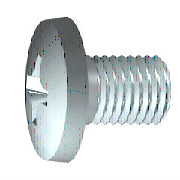
# Autodesk Inventor part: JIS B 1111 - M8x30
Saved by Autodesk Inventor 2022 (Build 260153000, 153)
## iProperties
Created: 2021-02-02
Part Number: JIS B 1111 - M8x30
Material: Сталь, мягкая
Description: Винты с низкой цилиндрической головкой
Document SubType Name: Modeling
Standard: JIS B 1111
Designer: Petrov Ivan
Standards Organization: JIS
Language: ru-RU
Size Designation: M8x30
Categories: <MemberInstance><Categories><Category DisplayName="Крепежные изделия" InternalName="e4da775c-781d-43d5-af7c-5136215cf5a6" Mnemonic="FSTN"><Category DisplayName="Болты  Винты" InternalName="536e6df0-f778-49ac-b2f2-25c71d2aa0b2" Mnemonic="SCRW"><CategoryParameter DisplayName="Обозначение номинального диаметра" InternalName="03caf894-eafd-4c09-a035-916ac084b87b" Mnemonic="nomdiadesig"/><CategoryParameter DisplayName="Номинальная длина" InternalName="238ecbaf-3e6c-45dd-aa95-4068c8e0fd02" Mnemonic="nomlen"/><CategoryParameter DisplayName="Обозначение резьбы" InternalName="586d5e89-370a-4089-914f-0110033585c7" Mnemonic="thrdesign"/><CategoryParameter DisplayName="Обозначение серии резьб" InternalName="87c5849c-b3a5-4c3e-9c9b-2feecef9be86" Mnemonic="thrserdsgn"/><CategoryParameter DisplayName="Номинальный диаметр" InternalName="8bbe3f8e-44cf-40a9-a251-3a6edc8168d6" Mnemonic="nomdia"/><CategoryParameter DisplayName="Тип резьбы" InternalName="b4bbb7bc-d6aa-4c9f-a9a9-4152b9f6fe49" Mnemonic="thrtype"/><CategoryParameter DisplayName="Шаг резьбы" InternalName="bb82302e-82d8-4176-8fc1-c5d7bb17d5ad" Mnemonic="pitch1"/><CategoryParameter DisplayName="Витков на единицу" InternalName="bdc6e7d2-ffd0-4d9c-a173-16b95ebb912d" Mnemonic="thrperunit1"/><CategoryParameter DisplayName="Класс резьбы" InternalName="ebc0d23b-2cc6-4d2a-b376-d52aae53bab6" Mnemonic="thrclss"/><Category DisplayName="С углублением под ключ" InternalName="55e06bf3-7e58-486c-bbdc-745fcc60664d" Mnemonic="CLSCRW"><CategoryParameter DisplayName="Диаметр стержня" InternalName="179dbae3-102f-48bb-85fe-1e3ecd34f7cc" Mnemonic="grpdia"/><CategoryParameter DisplayName="Длина резьбы" InternalName="3268731d-5f9a-4750-8b01-4a959c46fbf2" Mnemonic="thrlen"/><CategoryParameter DisplayName="Диаметр головки" InternalName="46177176-dbdd-4a1b-aefd-4c60c45016af" Mnemonic="headdia"/><CategoryParameter DisplayName="Длина стержня" InternalName="52eab69f-422f-4795-9995-175a1b827e67" Mnemonic="grplen"/><CategoryParameter DisplayName="Тип" InternalName="59a7e495-7a0c-4a5c-bdfd-c090c5f6e2db" Mnemonic="type"/><CategoryParameter DisplayName="Высота головки" InternalName="99c92c4c-4a02-4ebe-9e64-948fb169e19e" Mnemonic="headh"/></Category></Category></Category><Category DisplayName="ТипДанных" InternalName="23b78d0f-2648-40c6-8793-ca6db495c9e8" Mnemonic="DATATYPE"><CategoryParameter DisplayName="ОтображаемоеИмя" InternalName="05415f3d-3907-474b-a020-eb9d644f4cf3" Mnemonic="DISPLAYNAME"/><CategoryParameter DisplayName="Стандарт" InternalName="0c0a119c-1e12-4c84-803f-101930972f5e" Mnemonic="STANDARD"/><CategoryParameter DisplayName="Наименование" InternalName="13903e3d-64b1-4950-80da-f627842ea37f" Mnemonic="DESCRIPTION"/><CategoryParameter DisplayName="Обозначение" InternalName="2675968c-4ce5-49e0-a4f5-552d29089031" Mnemonic="DESIGNATION"/><CategoryParameter DisplayName="Строка по умолчанию" InternalName="2af9ec52-faaa-4026-b378-f9fa4afca842" Mnemonic="DEFAULTROW"/><CategoryParameter DisplayName="Имя папки" InternalName="3f06958e-8713-4116-9be7-ed6184ecc97b" Mnemonic="FOLDERNAME"/><CategoryParameter DisplayName="Указатель редакций" InternalName="45a75005-10b1-4dfc-8d6d-dfe629f0b93c" Mnemonic="REVISIONGUID"/><CategoryParameter DisplayName="ИмяФайла" InternalName="8b46a4cc-9585-4fed-90c3-899f57e09a73" Mnemonic="FILENAME"/><CategoryParameter DisplayName="ОргСтанд" InternalName="8f5914e1-4693-403f-8ab5-d37768198c9d" Mnemonic="STDSORG"/><CategoryParameter DisplayName="Версия семейства" InternalName="914462f6-6e19-4b14-ba84-155b9680b1d0" Mnemonic="FAMILYREVISION"/><CategoryParameter DisplayName="Редакция стандарта" InternalName="91d5a463-65c2-4fde-b823-3b7fea5e8e17" Mnemonic="STANDARDREVISION"/><CategoryParameter DisplayName="редакция элемента" InternalName="a65d44b9-392f-4f4f-857b-e4b3d54996fe" Mnemonic="MEMBERREVISION"/><CategoryParameter DisplayName="ФорматКлипа" InternalName="bc51e27b-3422-4e78-93ef-cec197ddf230" Mnemonic="CLIPFORMAT"/><CategoryParameter DisplayName="Изготовитель" InternalName="cd6c7a72-a28a-4e50-99a9-2c7f4e13e5ad" Mnemonic="MANUFACTURER"/><CategoryParameter DisplayName="ВнутреннееИмя" InternalName="cf1d0246-76d9-4b4a-8305-fa0409afb5c1" Mnemonic="INTERNALNAME"/><CategoryParameter DisplayName="Метрическая" InternalName="e2385c5b-1ea4-4823-96a8-8de651266ec3" Mnemonic="ISMETRIC"/><Category DisplayName="Деталь" InternalName="c0e0b642-3bcb-4cc8-9e80-f96d35c4afa4" Mnemonic="PART"><CategoryParameter DisplayName="Номер детали" InternalName="016b6077-bfbe-49bd-92c9-d8d59c39c941" Mnemonic="PARTNUMBER"/><CategoryParameter DisplayName="Инвентарный номер" InternalName="4dba7c1c-e26c-444e-836c-b08b433409a8" Mnemonic="STOCKNUMBER"/><CategoryParameter DisplayName="Ключ материала" InternalName="5c9a8adb-dd2b-4535-b97f-0a94a95fe41f" Mnemonic="MATERIALKEY"/><CategoryParameter DisplayName="Материал" InternalName="818a152a-d3c3-49ca-80ee-df7d91421b8e" Mnemonic="MATERIAL"/></Category></Category><Category DisplayName="Схема предыдущей версии DA" InternalName="924fff40-ddd0-4eff-ad42-30e3774ef79e" Mnemonic="LEGACYMAPDA"><CategoryParameter DisplayName="DACookie" InternalName="316934ee-8fe1-4c7a-9c36-f2d79e1add1a" Mnemonic="DACOOKIE"/></Category></Categories><FamilyTemplate Id="J11119"><FamilyTemplateParameters><FamilyTemplateParameter ObjectType="kUserParameterObject" ValueType="xs:double" Id="1" ObjectReferenceKey="NND"/><FamilyTemplateParameter ObjectType="kUserParameterObject" ValueType="xs:double" Id="2" ObjectReferenceKey="NLG"/><FamilyTemplateParameter ObjectType="kUserParameterObject" ValueType="xs:double" Id="3" ObjectReferenceKey="PTC"/><FamilyTemplateParameter ObjectType="kUserParameterObject" ValueType="xs:double" Id="4" ObjectReferenceKey="Dk"/><FamilyTemplateParameter ObjectType="kUserParameterObject" ValueType="xs:double" Id="5" ObjectReferenceKey="ParK"/><FamilyTemplateParameter ObjectType="kUserParameterObject" ValueType="xs:double" Id="6" ObjectReferenceKey="M"/><FamilyTemplateParameter ObjectType="kUserParameterObject" ValueType="xs:double" Id="7" ObjectReferenceKey="r"/><FamilyTemplateParameter ObjectType="kUserParameterObject" ValueType="xs:double" Id="8" ObjectReferenceKey="b"/><FamilyTemplateParameter ObjectType="kUserParameterObject" ValueType="xs:double" Id="9" ObjectReferenceKey="q"/><FamilyTemplateParameter ObjectType="kUserParameterObject" ValueType="xs:double" Id="10" ObjectReferenceKey="ParF"/><FamilyTemplateParameter ObjectType="kUserParameterObject" ValueType="xs:double" Id="117" ObjectReferenceKey="THREADDIA"/><FamilyTemplateParameter ObjectType="kPropertyObject" ValueType="xs:string" Id="100" ObjectReferenceKey="{32853F0F-3444-11d1-9E93-0060B03C1CA6}" SubObjectId="52"/><FamilyTemplateParameter ObjectType="kPropertyObject" ValueType="xs:string" Id="105" ObjectReferenceKey="{32853F0F-3444-11d1-9E93-0060B03C1CA6}" SubObjectId="5"/><FamilyTemplateParameter ObjectType="kPartComponentDefinitionObject" ValueType="xs:string" Id="110" SubObjectId="Material"/><FamilyTemplateParameter ObjectType="kThreadFeatureObject" ValueType="xs:structure" Id="300" ObjectReferenceKey="10020000100000000e120000000000008000000000000000" SubObjectId="ThreadInfo"><FamilyTemplateParameter ObjectType="" ValueType="xs:string" Id="301" SubObjectId="ThreadDesignation"/><FamilyTemplateParameter ObjectType="" ValueType="xs:string" Id="302" SubObjectId="ThreadType"/><FamilyTemplateParameter ObjectType="" ValueType="xs:string" Id="303" SubObjectId="ThreadClass"/></FamilyTemplateParameter></FamilyTemplateParameters></FamilyTemplate><CategoryParameterMap><ParamToTemplateMap><ParamToTemplate CategoryParameter="//CategoryParameter[@InternalName='05415f3d-3907-474b-a020-eb9d644f4cf3']" ConstantValue="JIS B 1111"/><ParamToTemplate CategoryParameter="//CategoryParameter[@InternalName='cf1d0246-76d9-4b4a-8305-fa0409afb5c1']" ConstantValue="129553A9-507D-4187-9D76-E3FDB36033EF"/><ParamToTemplate CategoryParameter="//CategoryParameter[@InternalName='3f06958e-8713-4116-9be7-ed6184ecc97b']" ConstantValue="JIS B 1111(1)"/><ParamToTemplate CategoryParameter="//CategoryParameter[@InternalName='914462f6-6e19-4b14-ba84-155b9680b1d0']" ConstantValue="10"/><ParamToTemplate CategoryParameter="//CategoryParameter[@InternalName='bc51e27b-3422-4e78-93ef-cec197ddf230']" ConstantValue="CF_INVENTOR.STDPARTS"/><ParamToTemplate CategoryParameter="//CategoryParameter[@InternalName='e2385c5b-1ea4-4823-96a8-8de651266ec3']" ConstantValue="true"/><ParamToTemplate CategoryParameter="//CategoryParameter[@InternalName='13903e3d-64b1-4950-80da-f627842ea37f']" ConstantValue="Binding head screws"/><ParamToTemplate CategoryParameter="//CategoryParameter[@InternalName='8f5914e1-4693-403f-8ab5-d37768198c9d']" ConstantValue="JIS"/><ParamToTemplate CategoryParameter="//CategoryParameter[@InternalName='0c0a119c-1e12-4c84-803f-101930972f5e']" ConstantValue="JIS B 1111"/><ParamToTemplate CategoryParameter="//CategoryParameter[@InternalName='cd6c7a72-a28a-4e50-99a9-2c7f4e13e5ad']" TemplateParameter="104"/><ParamToTemplate CategoryParameter="//CategoryParameter[@InternalName='91d5a463-65c2-4fde-b823-3b7fea5e8e17']" TemplateParameter="103"/><ParamToTemplate CategoryParameter="//CategoryParameter[@InternalName='45a75005-10b1-4dfc-8d6d-dfe629f0b93c']" ConstantValue="adaa1bef-3dad-41a7-8a06-32a4a9cd9839"/><ParamToTemplate CategoryParameter="//CategoryParameter[@InternalName='2af9ec52-faaa-4026-b378-f9fa4afca842']" ConstantValue="10"/><ParamToTemplate CategoryParameter="//CategoryParameter[@InternalName='8b46a4cc-9585-4fed-90c3-899f57e09a73']" ConstantValue="JIS B 1111 - M8x30(1)"/><ParamToTemplate CategoryParameter="//CategoryParameter[@InternalName='a65d44b9-392f-4f4f-857b-e4b3d54996fe']" ConstantValue="4721F653-DFC0-4489-BD95-3314774090E3"/><ParamToTemplate CategoryParameter="//CategoryParameter[@InternalName='52eab69f-422f-4795-9995-175a1b827e67']" ConstantValue="2,34"/><ParamToTemplate CategoryParameter="//CategoryParameter[@InternalName='03caf894-eafd-4c09-a035-916ac084b87b']" ConstantValue="M8"/><ParamToTemplate CategoryParameter="//CategoryParameter[@InternalName='316934ee-8fe1-4c7a-9c36-f2d79e1add1a']" ConstantValue="*JIS~J11119~M8x30~30*"/><ParamToTemplate CategoryParameter="//CategoryParameter[@InternalName='2675968c-4ce5-49e0-a4f5-552d29089031']" TemplateParameter="100"/><ParamToTemplate CategoryParameter="//CategoryParameter[@InternalName='46177176-dbdd-4a1b-aefd-4c60c45016af']" TemplateParameter="4"/><ParamToTemplate CategoryParameter="//CategoryParameter[@InternalName='818a152a-d3c3-49ca-80ee-df7d91421b8e']" TemplateParameter="110"/><ParamToTemplate CategoryParameter="//CategoryParameter[@InternalName='238ecbaf-3e6c-45dd-aa95-4068c8e0fd02']" TemplateParameter="2"/><ParamToTemplate CategoryParameter="//CategoryParameter[@InternalName='8bbe3f8e-44cf-40a9-a251-3a6edc8168d6']" TemplateParameter="1"/><ParamToTemplate CategoryParameter="//CategoryParameter[@InternalName='016b6077-bfbe-49bd-92c9-d8d59c39c941']" TemplateParameter="105"/><ParamToTemplate CategoryParameter="//CategoryParameter[@InternalName='bb82302e-82d8-4176-8fc1-c5d7bb17d5ad']" TemplateParameter="3"/><ParamToTemplate CategoryParameter="//CategoryParameter[@InternalName='99c92c4c-4a02-4ebe-9e64-948fb169e19e']" TemplateParameter="5"/><ParamToTemplate CategoryParameter="//CategoryParameter[@InternalName='ebc0d23b-2cc6-4d2a-b376-d52aae53bab6']" TemplateParameter="303"/><ParamToTemplate CategoryParameter="//CategoryParameter[@InternalName='586d5e89-370a-4089-914f-0110033585c7']" TemplateParameter="301"/><ParamToTemplate CategoryParameter="//CategoryParameter[@InternalName='b4bbb7bc-d6aa-4c9f-a9a9-4152b9f6fe49']" TemplateParameter="302"/><ParamToTemplate CategoryParameter="//CategoryParameter[@InternalName='3268731d-5f9a-4750-8b01-4a959c46fbf2']" TemplateParameter="8"/></ParamToTemplateMap></CategoryParameterMap></MemberInstance>
Density: 7.85 g/cm^3
Appearance: С умеренной полировкой
IsCustomPart: 0
Author: Petrov Ivan
Autodesk Inventor part; units mm, degrees
ref_plane "YZ Plane" through (0, 0, 0) normal (1, 0, 0) x (0, 1, 0)
sketch "Эскиз2" plane through (0, 0, 0) normal (0, 0, 1) x (1, 0, 0)
  circle A0 centre (0, 0) radius 3.375
  dimension "d3" = 6.75
extrude "Выдавливание1" add sketch "Эскиз2" against normal blind 2.34
sketch "Эскиз3" plane through (0, 0, -2.34) normal (0, 0, -1) x (-1, 0, 0)
  circle A0 centre (0, 0) radius 4
  circle A1 centre (0, 0) radius 3.375 construction
  dimension "d28" = 360
  dimension "d9" = 8
  constraints: 1 centre point, 1 concentric
  measures "d9" diameter of A0
extrude "Выдавливание2" add sketch "Эскиз3" along normal blind 27.66
chamfer "Фаска1" distance 0.625 distance2 0.625 1 edges at (4, 0, -2.34) measured on face at (-3.7202, -0.5883, -2.34)
sketch "Эскиз4" plane through (0, 0, 0) normal (0, 0, 1) x (1, 0, 0)
  circle A0 centre (0, 0) radius 8.2
  circle A1 centre (0, 0) radius 3.375 construction
  dimension "d15" = 16.4
  constraints: 1 centre point, 1 concentric
  measures "d15" diameter of A0
extrude "Выдавливание3" add sketch "Эскиз4" along normal blind 3.1
fillet "Сопряжение1" radius 0.4 1 edges at (-3.375, 0, 0)
sketch "Эскиз5" plane through (0, 0, 0) normal (0, 1, 0) x (-1, 0, 0)
  line L0 (8.2, 3.1) -> (8.2, 0)
  line L1 (7.9288, 3.1) -> (8.2, 3.1)
  line L2 (8.2, 0) -> (7.9288, 3.1)
  line L3 (-8.2, 3.1) -> (8.2, 3.1) construction
  line L4 (-8.2, 0) -> (8.2, 0) construction
  line L5 (0, -0.62) -> (0, 3.72) projected
  line L6 (11.48, 0) -> (-11.48, 0) projected
  dimension "d20" = 5
  dimension "d56" = 8.2
  dimension "d57" = 3.1
  constraints: 6 end point, 1 horizontal, 1 point on line, 1 vertical
  measures "d20" angle of L2 L0
  measures "d56" distance between parallel lines of L0 L5
  measures "d57" distance between parallel lines of L6 L1
revolve "Вращение1" cut sketch "Эскиз5" angle 360 about axis through (0, 0, -10) along (0, 0, 1)
sketch "Эскиз6" plane through (0, 0, 0) normal (0, 1, 0) x (-1, 0, 0)
  line L0 (0, 4.8) -> (0, 3.1)
  arc A0 (7.9288, 3.1) -> (0, 4.8) centre (-2.8592, -27.8751) ccw
  line L1 (0, 3.1) -> (7.9288, 3.1)
  line L2 (7.9288, 3.1) -> (-7.9288, 3.1) construction
  line L3 (0, -4.4495) -> (0, 0.4495)
  line L4 (0, -34.4594) -> (0, 11.6302) projected
  line L5 (11.1636, 0) -> (-11.1108, 0) projected
  dimension "d58" = 1.7
  dimension "d59" = 7.9288
  dimension "d60" = 0
  dimension "d62" = 32.8
  constraints: 6 end point, 2 point on circle, 1 centre point, 1 horizontal, 1 point on line, 1 vertical
  measures "d58" distance of L0.start L0.end
  measures "d59" distance of L0.end L1.end
  measures "d60" distance between parallel lines of L4 L0
  measures "d62" radius of A0
revolve "Вращение2" add sketch "Эскиз6" angle 360 about axis through (0, 0, -4.4495) along (0, 0, 1)
sketch "Эскиз7" plane through (0, 0, 0) normal (0, 1, 0) x (-1, 0, 0)
  line L0 (3.9, 4.8) -> (-3.9, 4.8)
  line L1 (1.8669, 0.44) -> (3.9, 4.8)
  line L2 (-1.8669, 0.44) -> (1.8669, 0.44)
  line L3 (-3.9, 4.8) -> (-1.8669, 0.44)
  line L4 (0, -0.432) -> (0, 5.672) projected
  line L5 (5.46, 0) -> (-5.46, 0) projected
  dimension "d32" = 4.36
  dimension "d34" = 65
  dimension "d36" = 65
  dimension "d63" = 3.9
  dimension "d64" = 4.8
  dimension "d65" = 7.8
  constraints: 8 end point, 2 horizontal
  measures "d32" vertical distance of L0.end L2.start
  measures "d34" angle of L3 L0
  measures "d36" angle of L0 L1
  measures "d63" distance from line of L4 L0.end
  measures "d64" distance between parallel lines of L5 L0
  measures "d65" distance of L0.start L0.end
extrude "Выдавливание4" cut sketch "Эскиз7" against normal mid plane 2.6
sketch "Эскиз8" plane through (0, 0, 0) normal (1, 0, 0) x (0, 1, 0)
  line L0 (-1.8669, 0.44) -> (-3.9, 4.8)
  line L1 (1.8669, 0.44) -> (-1.8669, 0.44)
  line L2 (3.9, 4.8) -> (1.8669, 0.44)
  line L3 (-3.9, 4.8) -> (3.9, 4.8)
  line L4 (0, -0.432) -> (0, 5.672) projected
  line L5 (-5.46, 0) -> (5.46, 0) projected
  dimension "d40" = 65
  dimension "d42" = 65
  dimension "d44" = 4.36
  dimension "d66" = 7.8
  dimension "d67" = 4.8
  dimension "d69" = 3.9
  constraints: 8 end point, 2 horizontal
  measures "d40" angle of L0 L3
  measures "d42" angle of L3 L2
  measures "d44" vertical distance of L0.end L0.start
  measures "d66" distance of L0.end L2.start
  measures "d67" distance between parallel lines of L5 L3
  measures "d69" distance from line of L4 L0.end
extrude "Выдавливание5" cut sketch "Эскиз8" along normal mid plane 2.6
sketch "Эскиз9" plane through (0, 0, 0) normal (0, 1, 0) x (-1, 0, 0)
  line L0 (0, 4.8) -> (0, 0.44)
  line L1 (3.12, 4.8) -> (0, 4.8)
  line L2 (0, 0.44) -> (3.12, 4.8)
  line L3 (-8.2, 0) -> (8.2, 0) construction
  line L4 (0, -0.96) -> (0, 5.76) projected
  line L5 (11.48, 0) -> (-11.48, 0) projected
  dimension "d50" = 4.36
  dimension "d52" = 4.36
  dimension "d54" = 3.12
  dimension "d70" = 0
  dimension "d71" = 4.8
  constraints: 6 end point, 1 vertical
  measures "d50" distance of L0.start L0.end
  measures "d52" vertical distance of L1.start L0.end
  measures "d54" distance of L1.start L0.start
  measures "d70" distance between parallel lines of L4 L0
  measures "d71" distance from line of L3 L1.start
revolve "Вращение3" cut sketch "Эскиз9" angle 360 about axis through (0, 0, -10) along (0, 0, 1)
thread "Резьба1" size "M8x1.25" class "6g" standard "ISO Metric profile" full length
ref_plane "MSC_PF1" through (0, 0, 0) normal (1, 0, 0) x (0, 1, 0)
ref_plane "MSC_PT1" through (0, 0, 0) normal (0, 0, -1) x (-1, 0, 0)
equation "\"d4\" = -b + NLG"
equation "\"d9\" = NND"
equation "\"d10\" = b"
equation "\"d12\" = -0.5 * msp_ds + 0.5 * NND"
equation "\"d13\" = 0.5 * NND - 0.5 * msp_ds"
equation "\"d15\" = Dk"
equation "\"d16\" = ParK"
equation "\"d18\" = r"
equation "\"d32\" = q"
equation "\"d63\" = 0.5 * M"
equation "\"d64\" = ParK + ParF"
equation "\"d65\" = M"
equation "\"d37\" = 2 * msp_s"
equation "\"d44\" = q"
equation "\"d66\" = M"
equation "\"d67\" = ParK + ParF"
equation "\"d69\" = 0.5 * M"
equation "\"d47\" = 2 * msp_s"
equation "\"d3\" = msp_ds"
equation "\"d56\" = 0.5 * Dk"
equation "\"d57\" = ParK"
equation "\"d58\" = ParF"
equation "\"d59\" = 0.5 * Dk - msp_v"
equation "\"d62\" = 2 * Dk"
equation "\"d50\" = q"
equation "\"d52\" = q"
equation "\"d54\" = msp_rr"
equation "\"d71\" = ParK + ParF"
equation "\"PTC\" = 1.25"
equation "\"NLG\" = 30"
equation "\"Dk\" = 16.4"
equation "\"ParK\" = 3.1"
equation "\"NND\" = 8"
equation "\"M\" = 7.8"
equation "\"q\" = 4.36"
equation "\"r\" = 0.4"
equation "\"msp_ds\" = NND - PTC"
equation "\"b\" = 27.66"
equation "\"msp_x\" = 1.25 * PTC"
equation "\"msp_s\" = 0.166667 * M"
equation "\"msp_rr\" = 0.4 * M"
equation "\"ParF\" = 1.7"
equation "\"msp_v\" = 0.0874887 * ParK"
equation "\"THREADDIA\" = NND"
body "Solid1"
